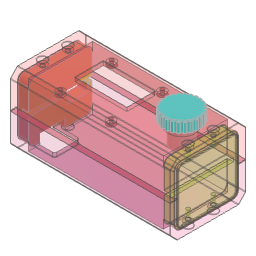
Gadget (Autodesk Fusion 360 design; units mm, degrees)
Autodesk Fusion 360 part; units mm, degrees
(part 1 of 2)
sketch "Top" plane through (0, 0, 0) normal (0, 0, 1) x (1, 0, 0) in component "Board"
  line L0 (35, 15) -> (-35, 15)
  line L1 (-35, 15) -> (-35, -15)
  line L2 (-35, -15) -> (35, -15)
  line L3 (35, -15) -> (35, 15)
  line L4 (35, 15) -> (-35, -15) construction
  line L5 (-35, 15) -> (35, -15) construction
  circle A0 centre (-33, -13) radius 1
  circle A1 centre (33, -13) radius 1
  circle A2 centre (-33, 13) radius 1
  circle A3 centre (33, 13) radius 1
  line L6 (6.5, -14.5) -> (-21, -14.5)
  line L7 (-21, -14.5) -> (-21, 13.3)
  line L8 (-21, 13.3) -> (6.5, 13.3)
  line L9 (6.5, 13.3) -> (6.5, -14.5)
  line L10 (6.5, -14.5) -> (-21, 13.3) construction
  line L11 (-21, -14.5) -> (6.5, 13.3) construction
  circle A4 centre (24, 1.5) radius 3
  line L12 (-21, 10.8) -> (6.5, 10.8)
  line L13 (15.5167, -1.5) -> (30.0322, -1.5) construction
  line L14 (21.3737, 2.95) -> (26.6263, 2.95)
  circle A5 centre (-19.25, -12.75) radius 1
  circle A6 centre (-19.25, -12.75) radius 1.75
  line L15 (-21, -0.6) -> (6.5, -0.6) construction
  line L16 (-7.25, -14.5) -> (-7.25, 13.3) construction
  circle A7 centre (4.75, -12.75) radius 1
  circle A8 centre (4.75, -12.75) radius 1.75
  circle A9 centre (-19.25, 11.55) radius 1.75
  circle A10 centre (-19.25, 11.55) radius 1
  circle A11 centre (4.75, 11.55) radius 1
  circle A12 centre (4.75, 11.55) radius 1.75
  line L17 (-21, -10.5) -> (6.5, -10.5)
  line L18 (-21, 9.3) -> (6.5, 9.3)
  point P0 (-7.25, -0.6)
  dimension "d1" = 70
  dimension "d2" = 30
  dimension "d3" = 2
  dimension "d4" = 2
  dimension "d5" = 2
  dimension "d8" = 66
  dimension "d9" = 26
  dimension "d10" = 27.5
  dimension "d11" = 27.8
  dimension "d12" = 14
  dimension "d13" = 0.5
  dimension "d14" = 6
  dimension "d15" = 13.5
  dimension "d16" = 11
  dimension "d29" = 2.5
  dimension "d36" = 4.45
  dimension "d40" = 2
  dimension "d41" = 3.5
  dimension "d42" = 4
  dimension "d43" = 4
  constraint horizontal L0
  constraint perpendicular L0 L1
  constraint parallel L0 L2
  constraint parallel L1 L3
  constraint coincident L4 origin
  constraint coincident L5 origin
  constraint horizontal L6
  constraint perpendicular L6 L7
  constraint parallel L6 L8
  constraint parallel L7 L9
  constraint coincident L10 P0
  constraint coincident L11 P0
  constraint coincident L7 L12.start
  constraint coincident L9 L12.end
  constraint perpendicular L9 L12
  constraint horizontal L13
  constraint tangent A4 L13
  constraint coincident A4 L14.start
  constraint coincident A4 L14.end
  constraint horizontal L14
  constraint concentric A5 A6
  constraint tangent L7 A6
  constraint tangent L6 A6
  constraint midpoint L7 L15.start
  constraint midpoint L9 L15.end
  constraint midpoint L6 L16.start
  constraint midpoint L8 L16.end
  constraint symmetric A5 L16 A7
  constraint symmetric A6 L16 A8
  constraint symmetric A5 L15 A10
  constraint symmetric A6 L15 A9
  constraint symmetric L15 A7 A11
  constraint symmetric L15 A8 A12
  constraint coincident L7 L17.start
  constraint coincident L9 L17.end
  constraint perpendicular L9 L17
  constraint coincident L7 L18.start
  constraint coincident L9 L18.end
  constraint perpendicular L9 L18
  measures "d1" distance of L1.end L2.end
  measures "d2" distance of L0.end L1.end
  measures "d3" diameter of A0
  measures "d4" distance of L1 A0.centre
  measures "d5" distance of L2 A0.centre
  measures "d10" distance of L7.end L8.end
  measures "d11" distance of L6.end L7.end
  measures "d12" distance of L1 L7
  measures "d13" distance of L2 L6
  measures "d14" diameter of A4
  measures "d15" distance of L0 A4.centre
  measures "d16" distance of L3 A4.centre
  measures "d29" distance of L7.end L12.start
  measures "d36" distance of L13 L14.end
  measures "d40" diameter of A5
  measures "d41" diameter of A6
  measures "d42" distance of L6.start L17.end
  measures "d43" distance of L8.end L18.end
extrude "Extrude1" add sketch "Top" along normal mid plane 1.6 contours L0 L1 L2 L3 | L6 L9 A8 | L6 L7 L9 A6 A8 L17 | A8 | L6 L7 A6 | A6 | L7 L9 L17 L18 | L7 L9 L12 A9 A12 L18 | L9 L12 A12 | L8 L9 A12 | L12 A11 A12 | L12 A11 A12 | L7 L12 A9 | L8 L12 A9 A12 | L12 A11 | L12 A11 | L7 L8 A9 | L12 A9 A10 | L12 A9 A10 | L12 A10 | L12 A10 | A4 L14 | A4 L14 | A5 | A7 makes body 1 in component "Board"
extrude "Extrude2" add sketch "Top" along normal blind 14.5 from surface at 0.8 contours L6 L9 A8 | L6 L7 L9 A6 A8 L17 | A8 | L6 L7 A6 | A6 | L7 L9 L17 L18 | L7 L9 L12 A9 A12 L18 | L9 L12 A12 | L8 L9 A12 | L12 A11 A12 | L12 A11 A12 | L7 L12 A9 | L8 L12 A9 A12 | L7 L8 A9 | L12 A9 A10 | L12 A9 A10 bodies 1 in component "Board"
extrude "Extrude4" cut sketch "Top" along normal up to surface (10.7 mm away) from surface at 0.8 contours L6 L9 A8 | L6 L7 L9 A6 A8 L17 | A8 | L6 L7 A6 | A6 | L7 L9 L17 L18 | L7 L9 L12 A9 A12 L18 | L12 A11 A12 | L12 A11 | L12 A9 A10 | L12 A10 | A5 | A7 picked at (5.7851, 10.4689) picked at (4.9322, 10.7708) picked at (-18.2149, 10.4689) picked at (-19.4322, 10.7708) bodies 1 in component "Board"
extrude "Extrude7" cut sketch "Top" along normal through all from surface at 13.5 contours L6 L9 A8 | L6 L7 L9 A6 A8 L17 | A8 | L6 L7 A6 | A6 | L7 L9 L12 A9 A12 L18 | L9 L12 A12 | L8 L9 A12 | L12 A11 A12 | L12 A11 A12 | L7 L12 A9 | L8 L12 A9 A12 | L7 L8 A9 | L12 A9 A10 | L12 A9 A10 bodies 1 in component "Board"
extrude "Extrude5" add sketch "Top" along normal blind 14.1 from surface at 0.8 contours A4 L14 | A4 L14 bodies 1 in component "Board"
extrude "Extrude6" cut sketch "Top" against normal blind 10 from surface at 14.9 contours A4 L14 picked at (23.2953, 3.1762) bodies 1 in component "Board"
sketch "Bottom" plane through (0, 0, 0) normal (0, 0, 1) x (1, 0, 0) in component "Board"
  line L0 (-35, -15) -> (35, -15) construction
  circle A0 centre (-33, -13) radius 1 construction
  line L1 (-35, 15) -> (-35, -15) construction
  line L2 (35, 15) -> (-35, 15) construction
  circle A1 centre (-33, 13) radius 1 construction
  circle A2 centre (33, 13) radius 1 construction
  line L3 (35, -15) -> (35, 15) construction
  circle A3 centre (33, -13) radius 1 construction
  line L4 (31.8, 12.7) -> (12.6, 12.7)
  line L5 (12.6, 12.7) -> (12.6, -13.5)
  line L6 (12.6, -13.5) -> (31.8, -13.5)
  line L7 (31.8, -13.5) -> (31.8, 12.7)
  line L8 (31.8, 12.7) -> (12.6, -13.5) construction
  line L9 (12.6, 12.7) -> (31.8, -13.5) construction
  line L10 (10.4, 14.8) -> (-2.8, 14.8)
  line L11 (-2.8, 14.8) -> (-2.8, -12.7)
  line L12 (-2.8, -12.7) -> (10.4, -12.7)
  line L13 (10.4, -12.7) -> (10.4, 14.8)
  line L14 (10.4, 14.8) -> (-2.8, -12.7) construction
  line L15 (-2.8, 14.8) -> (10.4, -12.7) construction
  line L16 (-10.8, 5.08) -> (-32, 5.08)
  line L17 (-32, 5.08) -> (-32, -12.7)
  line L18 (-32, -12.7) -> (-10.8, -12.7)
  line L19 (-10.8, -12.7) -> (-10.8, 5.08)
  line L20 (-10.8, 5.08) -> (-32, -12.7) construction
  line L21 (-32, 5.08) -> (-10.8, -12.7) construction
  line L22 (-25.9, 0.69) -> (-33.4, 0.69)
  line L23 (-33.4, 0.69) -> (-33.4, -8.31)
  line L24 (-33.4, -8.31) -> (-25.9, -8.31)
  line L25 (-25.9, -8.31) -> (-25.9, 0.69)
  line L26 (-25.9, 0.69) -> (-33.4, -8.31) construction
  line L27 (-33.4, 0.69) -> (-25.9, -8.31) construction
  line L28 (-29.65, -3.81) -> (-21.4, -3.81) construction
  line L29 (-31.5, 13) -> (-38.5, 13)
  line L30 (-38.5, 13) -> (-38.5, 4)
  line L31 (-38.5, 4) -> (-31.5, 4)
  line L32 (-31.5, 4) -> (-31.5, 13)
  line L33 (-31.5, 13) -> (-38.5, 4) construction
  line L34 (-38.5, 13) -> (-31.5, 4) construction
  point P0 (22.2, -0.4)
  point P1 (3.8, 1.05)
  point P2 (-21.4, -3.81)
  point P3 (-29.65, -3.81)
  point P4 (-35, 8.5)
  dimension "d46" = 19.2
  dimension "d47" = 26.2
  dimension "d48" = 1.5
  dimension "d49" = 3.2
  dimension "d50" = 13.2
  dimension "d51" = 27.5
  dimension "d53" = 2.2
  dimension "d54" = 8
  dimension "d55" = 17.78
  dimension "d56" = 21.2
  dimension "d57" = 7.5
  dimension "d58" = 9
  dimension "d59" = 1.4
  dimension "d70" = 63.8
  dimension "d378" = 7
  dimension "d379" = 9
  dimension "d400" = 2.3
  dimension "d401" = 2
  dimension "d402" = 2.3
  constraint horizontal L4
  constraint perpendicular L4 L5
  constraint parallel L4 L6
  constraint parallel L5 L7
  constraint coincident L8 P0
  constraint coincident L9 P0
  constraint horizontal L10
  constraint perpendicular L10 L11
  constraint parallel L10 L12
  constraint parallel L11 L13
  constraint coincident L14 P1
  constraint coincident L15 P1
  constraint horizontal L16
  constraint perpendicular L16 L17
  constraint parallel L16 L18
  constraint parallel L17 L19
  constraint coincident L20 P2
  constraint coincident L21 P2
  constraint horizontal L22
  constraint perpendicular L22 L23
  constraint parallel L22 L24
  constraint parallel L23 L25
  constraint coincident L26 P3
  constraint coincident L27 P3
  constraint coincident P3 L28.start
  constraint coincident P2 L28.end
  constraint perpendicular L17 L28
  constraint horizontal L29
  constraint perpendicular L29 L30
  constraint parallel L29 L31
  constraint parallel L30 L32
  constraint coincident L33 P4
  constraint coincident L34 P4
  constraint coincident L1 P4
  measures "d46" distance of L5.end L6.end
  measures "d47" distance of L4.end L5.end
  measures "d48" distance of L0 L6
  measures "d49" distance of L3 L7
  measures "d50" distance of L11.end L12.end
  measures "d51" distance of L10.end L11.end
  measures "d53" distance of L5 L13
  measures "d54" distance of L11 L19
  measures "d55" distance of L16.end L17.end
  measures "d56" distance of L17.end L18.end
  measures "d57" distance of L23.end L24.end
  measures "d58" distance of L22.end L23.end
  measures "d59" distance of L17 L22.end
  measures "d70" horizontal distance of L4.start L16.end
  measures "d378" distance of L30.end L31.end
  measures "d379" distance of L29.end L30.end
  measures "d400" distance of L0 L18
  measures "d401" distance of L2 L29
  measures "d402" distance of L0 L12
extrude "Extrude8" add sketch "Bottom" against normal blind 4 from surface at -0.8 contours L16 L17 L31 L32 | L16 L17 L29 L30 L31 L32 bodies 1 in component "Board"
extrude "Extrude9" add sketch "Bottom" against normal blind 13.5 from surface at -0.8 contours L16 L17 L18 L19 L22 L24 L25 L31 L32 | L16 L17 L31 L32 | L17 L22 L24 L25 bodies 1 in component "Board"
extrude "Extrude10" add sketch "Bottom" against normal blind 3.2 from surface at -12.7 contours L17 L22 L23 L24 | L17 L22 L24 L25 bodies 1 in component "Board"
extrude "Extrude11" add sketch "Bottom" against normal blind 13.9 from surface at -0.8 contours L10 L11 L12 L13 bodies 1 in component "Board"
extrude "Extrude12" add sketch "Bottom" against normal blind 13.9 from surface at -0.8 contours L4 L5 L6 L7 bodies 1 in component "Board"
sketch "Sketch1" plane through (0, 0, 0) normal (1, 0, 0) x (0, 1, 0) in component "Right"
  line L0 (12, -13.9) -> (-12, -13.9)
  line L1 (-15, -10.9) -> (-15, 10.9)
  line L2 (-12, 13.9) -> (12, 13.9)
  line L3 (15, 10.9) -> (15, -10.9)
  line L4 (15, -13.9) -> (-15, 13.9) construction
  line L5 (-15, -13.9) -> (15, 13.9) construction
  arc A0 (-12, 13.9) -> (-15, 10.9) centre (-12, 10.9) ccw
  arc A1 (15, 10.9) -> (12, 13.9) centre (12, 10.9) ccw
  arc A2 (12, -13.9) -> (15, -10.9) centre (12, -10.9) ccw
  arc A3 (-15, -10.9) -> (-12, -13.9) centre (-12, -10.9) ccw
  line L6 (-15, -0.9) -> (15, -0.9)
  line L7 (-15, 0.9) -> (15, 0.9)
  arc A4 (13.9, 10.9) -> (12, 12.8) centre (12, 10.9) ccw
  line L8 (-12, 12.8) -> (12, 12.8)
  arc A5 (-12, 12.8) -> (-13.9, 10.9) centre (-12, 10.9) ccw
  line L9 (-13.9, -10.9) -> (-13.9, 10.9)
  arc A6 (-13.9, -10.9) -> (-12, -12.8) centre (-12, -10.9) ccw
  line L10 (12, -12.8) -> (-12, -12.8)
  arc A7 (12, -12.8) -> (13.9, -10.9) centre (12, -10.9) ccw
  line L11 (13.9, 10.9) -> (13.9, -10.9)
  dimension "d192" = 30
  dimension "d193" = 27.8
  dimension "d194" = 3
  dimension "d209" = 1.1
  dimension "d393" = 1.8
  dimension "d394" = 0.9
  constraint horizontal L0
  constraint perpendicular L0 L1
  constraint parallel L0 L2
  constraint parallel L1 L3
  constraint coincident L4 origin
  constraint coincident L5 origin
  constraint coincident L4.end L1
  constraint coincident L4.end L2
  constraint tangent L1 A0
  constraint tangent L2 A0
  constraint coincident L5.end L3
  constraint coincident L5.end L2
  constraint tangent L3 A1
  constraint tangent L2 A1
  constraint equal A0 A1
  constraint coincident L4.start L0
  constraint coincident L4.start L3
  constraint tangent L0 A2
  constraint tangent L3 A2
  constraint equal A0 A2
  constraint coincident L5.start L0
  constraint coincident L5.start L1
  constraint tangent L0 A3
  constraint tangent L1 A3
  constraint equal A0 A3
  constraint coincident L1 L6.start
  constraint coincident L3 L6.end
  constraint perpendicular L3 L6
  constraint coincident L1 L7.start
  constraint coincident L3 L7.end
  constraint perpendicular L3 L7
  measures "d192" distance of L4.end L5.end
  measures "d193" distance of L5.start L4.end
  measures "d194" radius of A0
  measures "d393" distance of L6.end L7.end
  measures "d394" distance of origin L6
extrude "Extrude1'" add sketch "Sketch1" along normal blind 6 from surface at 32 separate body makes body 2 in component "Right"
extrude "Extrude2'" cut sketch "Sketch1" along normal blind 35 contours L3 L6 L7 L11 | L1 L6 L7 L9 | L6 L7 L9 L11 bodies 2 in component "Right"
extrude "Extrude5'" cut sketch "Sketch1" against normal blind 1 from surface at 38 contours L0 L1 L3 A2 A3 L6 L9 A6 L10 A7 L11 | L3 L6 L7 L11 | L1 L6 L7 L9 | L1 L2 L3 A0 A1 L7 A4 L8 A5 L9 L11 bodies 2 in component "Right"
sketch "Sketch2" plane through (0, 0, 13.9) normal (0, 0, 1) x (-1, 0, 0) in component "Right"
  line L0 (-32, -12) -> (-32, 12)
  line L1 (-32, 12) -> (-37, 12)
  line L2 (-37, -12) -> (-32, -12)
  line L3 (0, 0) -> (-32, 0) construction
  line L4 (-32, 0) -> (-37, 0) construction
  line L5 (-34.5, 0) -> (-34.5, -6) construction
  circle A0 centre (-34.5, -6) radius 0.875
  circle A1 centre (-34.5, 6) radius 0.875
  line L6 (-37, 12) -> (-37, -12)
  dimension "d202" = 6
  dimension "d203" = 1.75
  constraint coincident L3.start origin
  constraint midpoint L0 L3.end
  constraint midpoint L4 L5.start
  constraint perpendicular L4 L5
  constraint coincident L5.end A0.centre
  constraint symmetric L4 A0 A1
  constraint midpoint L4.end L6
  measures "d202" distance of L5.start L5.end
  measures "d203" diameter of A0
extrude "Extrude3" cut sketch "Sketch2" against normal blind 4 contours A0 | A1 bodies 2 in component "Right"
extrude "Extrude4'" cut sketch "Sketch2" along normal blind 4 from surface at -27.8 contours A0 | A1 bodies 2 in component "Right"
chamfer "Chamfer1" distance 0.2 angle 45 8 edges at (37, 0, 13.9) (37, 14.1213, 13.0213) (37, 15, 0) (37, 14.1213, -13.0213) (37, 0, -13.9) (37, -14.1213, -13.0213) (37, -15, 0) (37, -14.1213, 13.0213) 2 faces at (32, -4, -5.2333) (32, -4, 5.2333) on bodies 2 in component "Right"
sketch "Sketch1 (2)" plane through (0, 0, 0) normal (1, 0, 0) x (0, 1, 0) in component "Left"
  line L0 (12, -13.9) -> (-12, -13.9)
  line L1 (-15, -10.9) -> (-15, 10.9)
  line L2 (-12, 13.9) -> (12, 13.9)
  line L3 (15, 10.9) -> (15, -10.9)
  line L4 (15, -13.9) -> (-15, 13.9) construction
  line L5 (-15, -13.9) -> (15, 13.9) construction
  arc A0 (-12, 13.9) -> (-15, 10.9) centre (-12, 10.9) ccw
  arc A1 (15, 10.9) -> (12, 13.9) centre (12, 10.9) ccw
  arc A2 (12, -13.9) -> (15, -10.9) centre (12, -10.9) ccw
  arc A3 (-15, -10.9) -> (-12, -13.9) centre (-12, -10.9) ccw
  arc A4 (13.9, 10.9) -> (12, 12.8) centre (12, 10.9) ccw
  line L6 (-12, 12.8) -> (12, 12.8)
  arc A5 (-12, 12.8) -> (-13.9, 10.9) centre (-12, 10.9) ccw
  line L7 (-13.9, -10.9) -> (-13.9, 10.9)
  arc A6 (-13.9, -10.9) -> (-12, -12.8) centre (-12, -10.9) ccw
  line L8 (12, -12.8) -> (-12, -12.8)
  arc A7 (12, -12.8) -> (13.9, -10.9) centre (12, -10.9) ccw
  line L9 (13.9, 10.9) -> (13.9, -10.9)
  line L10 (-15, -0.9) -> (15, -0.9)
  line L11 (-15, 0.9) -> (15, 0.9)
  line L12 (2.19, -18.3) -> (-9.81, -18.3)
  line L13 (-9.81, -18.3) -> (-9.81, -10.3)
  line L14 (-9.81, -10.3) -> (2.19, -10.3)
  line L15 (2.19, -10.3) -> (2.19, -18.3)
  line L16 (2.19, -18.3) -> (-9.81, -10.3) construction
  line L17 (-9.81, -18.3) -> (2.19, -10.3) construction
  line L18 (4, -0.8) -> (13, -0.8)
  line L19 (13, -0.8) -> (13, -4.8)
  line L20 (13, -4.8) -> (4, -4.8)
  line L21 (4, -4.8) -> (4, -0.8)
  line L22 (3, -5.8) -> (3, 0.2)
  line L23 (3, 0.2) -> (14, 0.2)
  line L24 (14, 0.2) -> (14, -5.8)
  line L25 (14, -5.8) -> (3, -5.8)
  line L26 (-8.31, -12.7) -> (0.69, -12.7)
  line L27 (0.69, -12.7) -> (0.69, -15.9)
  line L28 (0.69, -15.9) -> (-8.31, -15.9)
  line L29 (-8.31, -15.9) -> (-8.31, -12.7)
  line L30 (-3.81, -14.3) -> (-8.31, -14.3) construction
  line L31 (-3.81, -14.3) -> (-3.81, -15.9) construction
  point P0 (-3.81, -14.3)
  dimension "d214" = 30
  dimension "d215" = 27.8
  dimension "d216" = 3
  dimension "d217" = 1.1
  dimension "d218" = 0.9
  dimension "d231" = 12
  dimension "d232" = 8
  dimension "d381" = -1
  dimension "d395" = 1.8
  constraint horizontal L0
  constraint perpendicular L0 L1
  constraint parallel L0 L2
  constraint parallel L1 L3
  constraint coincident L4 origin
  constraint coincident L5 origin
  constraint coincident L4.end L1
  constraint coincident L4.end L2
  constraint tangent L1 A0
  constraint tangent L2 A0
  constraint coincident L5.end L3
  constraint coincident L5.end L2
  constraint tangent L3 A1
  constraint tangent L2 A1
  constraint equal A0 A1
  constraint coincident L4.start L0
  constraint coincident L4.start L3
  constraint tangent L0 A2
  constraint tangent L3 A2
  constraint equal A0 A2
  constraint coincident L5.start L0
  constraint coincident L5.start L1
  constraint tangent L0 A3
  constraint tangent L1 A3
  constraint equal A0 A3
  constraint coincident L1 L10.start
  constraint coincident L3 L10.end
  constraint perpendicular L3 L10
  constraint coincident L1 L11.start
  constraint coincident L3 L11.end
  constraint perpendicular L3 L11
  constraint horizontal L12
  constraint perpendicular L12 L13
  constraint parallel L12 L14
  constraint parallel L13 L15
  constraint coincident L16 P0
  constraint coincident L17 P0
  constraint coincident P0 L30.start
  constraint coincident L29 L30.end
  constraint perpendicular L29 L30
  constraint midpoint L29 L30.end
  constraint coincident L28 L31.end
  constraint perpendicular L28 L31
  constraint midpoint L28 L31.end
  measures "d214" distance of L4.end L5.end
  measures "d215" distance of L5.start L4.end
  measures "d216" radius of A0
  measures "d218" vertical distance of origin L10.end
  measures "d231" distance of L13.end L14.end
  measures "d232" distance of L12.end L13.end
  measures "d395" distance of L10.end L11.end
extrude "Extrude1''" add sketch "Sketch1 (2)" against normal blind 6 from surface at -32 separate body contours L0 L3 A2 L8 A7 L9 L10 L15 L24 L25 | L7 A6 L8 A7 L9 L10 L13 L14 L15 L22 L25 | L3 L9 L10 L11 L23 L24 | L1 L2 L3 A0 A1 A4 L6 A5 L7 L9 L11 | L9 L10 L24 L25 | L9 L10 L23 L24 | L0 L1 A3 L7 A6 L8 L10 L13 | A4 L6 A5 L7 L9 L11 | L7 L9 L10 L11 L22 L23 | L9 L10 L18 L19 L21 L22 L23 | L9 L10 L19 L20 L21 L22 L25 | L1 L7 L10 L11 makes body 3 in component "Left"
extrude "Extrude2''" cut sketch "Sketch1 (2)" against normal blind 35 contours L3 L9 L10 L11 L23 L24 | L9 L10 L23 L24 | L7 L9 L10 L11 L22 L23 | L9 L10 L18 L19 L21 L22 L23 | L1 L7 L10 L11 | L10 L18 L19 L21 bodies 3 in component "Left"
extrude "Extrude3'" cut sketch "Sketch1 (2)" along normal blind 1 from surface at -38 contours L0 L3 A2 L8 A7 L9 L10 L15 L24 L25 | L0 L8 L15 L27 | L0 L8 L27 L29 | L3 L9 L10 L11 L23 L24 | L0 L8 L13 L29 | L1 L2 L3 A0 A1 A4 L6 A5 L7 L9 L11 | L9 L10 L24 L25 | L9 L10 L23 L24 | L0 L1 A3 L7 A6 L8 L10 L13 | L1 L7 L10 L11 bodies 3 in component "Left"
extrude "Extrude7'" cut sketch "Sketch1 (2)" along normal blind 1 from surface at -38 contours L9 L10 L24 L25 | L9 L10 L23 L24 | L9 L10 L18 L19 L21 L22 L23 | L9 L10 L19 L20 L21 L22 L25 bodies 3 in component "Left"
fillet "Fillet1" radius 1 2 edges at (-37.5, 3, 0.2) (-37.5, 3, -5.8) on bodies 3 in component "Left"
fillet "Fillet2" radius 1 5 edges at (-37, 8.95, -5.8) (-37, 3.2929, -5.5071) (-37, 3, -2.8) (-37, 3.2929, -0.0929) (-37, 8.95, 0.2) on bodies 3 in component "Left"
sketch "Sketch2 (2)" plane through (0, 0, 13.9) normal (0, 0, 1) x (-1, 0, 0) in component "Left"
  line L0 (37, -12) -> (37, 12)
  line L1 (37, 12) -> (32, 12)
  line L2 (32, 12) -> (32, -12)
  line L3 (32, -12) -> (37, -12)
  line L4 (0, 0) -> (32, 0) construction
  line L5 (32, 0) -> (37, 0) construction
  line L6 (34.5, 0) -> (34.5, -6) construction
  circle A0 centre (34.5, -6) radius 0.875
  circle A1 centre (34.5, 6) radius 0.875
  dimension "d235" = 5
  dimension "d236" = 6
  dimension "d237" = 1.75
  constraint coincident L4.start origin
  constraint midpoint L2 L4.end
  constraint perpendicular L0 L5
  constraint midpoint L5 L6.start
  constraint perpendicular L5 L6
  constraint coincident L6.end A0.centre
  constraint symmetric L5 A0 A1
  measures "d235" distance of L4.end L5.end
  measures "d236" distance of L6.start L6.end
  measures "d237" diameter of A0
extrude "Extrude4''" cut sketch "Sketch2 (2)" against normal blind 4 contours A0 | A1 bodies 3 in component "Left"
extrude "Extrude5''" cut sketch "Sketch2 (2)" along normal blind 4 from surface at -27.8 contours A0 bodies 3 in component "Left"
chamfer "Chamfer1'" distance 0.2 angle 45 9 edges at (-37, -14.1213, 13.0213) (-37, 0, 13.9) (-37, 14.1213, 13.0213) (-37, 15, 0) (-37, 14.1213, -13.0213) (-37, 7.095, -13.9) (-37, -10.905, -13.9) (-37, -14.1213, -13.0213) (-37, -15, 0) 2 faces at (-32, -4, 5.2333) (-32, -6.9367, -4.0333) on bodies 3 in component "Left"
sketch "Sketch1 (3)" plane through (0, 0, 0) normal (1, 0, 0) x (0, 1, 0) in component "Bottom"
  line L0 (-12, -13.9) -> (12, -13.9) construction
  line L1 (15, -10.9) -> (15, 10.9) construction
  line L2 (12, 13.9) -> (-12, 13.9) construction
  line L3 (-15, 10.9) -> (-15, -10.9) construction
  line L4 (-15, -13.9) -> (15, 13.9) construction
  line L5 (15, -13.9) -> (-15, 13.9) construction
  arc A0 (15, 10.9) -> (12, 13.9) centre (12, 10.9) ccw construction
  arc A1 (-12, 13.9) -> (-15, 10.9) centre (-12, 10.9) ccw construction
  arc A2 (-15, -10.9) -> (-12, -13.9) centre (-12, -10.9) ccw construction
  arc A3 (12, -13.9) -> (15, -10.9) centre (12, -10.9) ccw construction
  line L6 (-12, -13.1) -> (12, -13.1)
  arc A4 (12, -13.1) -> (14.2, -10.9) centre (12, -10.9) ccw
  line L7 (14.2, -10.9) -> (14.2, 10.9)
  arc A5 (14.2, 10.9) -> (12, 13.1) centre (12, 10.9) ccw
  line L8 (12, 13.1) -> (-12, 13.1)
  arc A6 (-12, 13.1) -> (-14.2, 10.9) centre (-12, 10.9) ccw
  line L9 (-14.2, 10.9) -> (-14.2, -10.9)
  arc A7 (-14.2, -10.9) -> (-12, -13.1) centre (-12, -10.9) ccw
  line L10 (-12, -14.1) -> (12, -14.1)
  arc A8 (12, -14.1) -> (15.2, -10.9) centre (12, -10.9) ccw
  line L11 (15.2, -10.9) -> (15.2, 10.9)
  arc A9 (15.2, 10.9) -> (12, 14.1) centre (12, 10.9) ccw
  line L12 (12, 14.1) -> (-12, 14.1)
  arc A10 (-12, 14.1) -> (-15.2, 10.9) centre (-12, 10.9) ccw
  line L13 (-15.2, 10.9) -> (-15.2, -10.9)
  arc A11 (-15.2, -10.9) -> (-12, -14.1) centre (-12, -10.9) ccw
  line L14 (-18, 10.9) -> (-18, -10.9)
  arc A12 (-18, -10.9) -> (-12, -16.9) centre (-12, -10.9) ccw construction
  line L15 (-12, -16.9) -> (12, -16.9)
  arc A13 (12, -16.9) -> (18, -10.9) centre (12, -10.9) ccw construction
  line L16 (18, -10.9) -> (18, 10.9)
  arc A14 (18, 10.9) -> (12, 16.9) centre (12, 10.9) ccw
  line L17 (12, 16.9) -> (-12, 16.9)
  arc A15 (-12, 16.9) -> (-18, 10.9) centre (-12, 10.9) ccw
  line L18 (18, 0) -> (-18, 0)
  line L19 (2.19, -18.3) -> (-9.81, -18.3)
  line L20 (2.19, -10.3) -> (2.19, -18.3)
  line L21 (-9.81, -18.3) -> (-9.81, -10.3)
  line L22 (-9.81, -10.3) -> (2.19, -10.3)
  line L23 (-15.2, -10.9) -> (-15.2, -15)
  line L24 (-15.2, -15) -> (15.2, -15)
  line L25 (15.2, -15) -> (15.2, -10.9)
  line L26 (-14.5804, -16.9) -> (-18, -13.2912)
  line L27 (-18, -13.2912) -> (-18, -10.9)
  line L28 (-14.5804, -16.9) -> (-12, -16.9)
  line L29 (-15, -13.9) -> (-16.2902, -15.0956) construction
  line L30 (0, 0) -> (0, -13.1) construction
  line L31 (14.5804, -16.9) -> (12, -16.9)
  line L32 (14.5804, -16.9) -> (18, -13.2912)
  line L33 (18, -13.2912) -> (18, -10.9)
  dimension "d244" = 30
  dimension "d245" = 27.8
  dimension "d246" = 3
  dimension "d247" = 3
  dimension "d248" = 3
  dimension "d249" = 3
  dimension "d250" = 0.2
  dimension "d251" = -0.8
  dimension "d252" = 3
  dimension "d284" = 15
  constraint horizontal L0
  constraint perpendicular L0 L1
  constraint parallel L0 L2
  constraint parallel L1 L3
  constraint coincident L4 L30.start
  constraint coincident L5 L30.start
  constraint coincident L30.start origin
  constraint coincident L4.end L2
  constraint coincident L4.end L1
  constraint tangent L2 A0
  constraint tangent L1 A0
  constraint coincident L5.end L2
  constraint coincident L5.end L3
  constraint tangent L2 A1
  constraint tangent L3 A1
  constraint coincident L4.start L0
  constraint coincident L4.start L3
  constraint tangent L0 A2
  constraint tangent L3 A2
  constraint coincident L5.start L0
  constraint coincident L5.start L1
  constraint tangent L0 A3
  constraint tangent L1 A3
  constraint midpoint L16 L18.start
  constraint midpoint L14 L18.end
  constraint perpendicular L14 L18
  constraint tangent A11 L23
  constraint parallel L13 L23
  constraint perpendicular L20 L24
  constraint perpendicular L24 L25
  constraint parallel L15 L28
  constraint parallel L14 L27
  constraint tangent A12 L26
  constraint coincident L26 L29.end
  constraint parallel L4 L29
  constraint midpoint L26 L29.end
  constraint midpoint L6 L30.end
  constraint perpendicular L6 L30
  constraint symmetric L14.end L30 A13.end
  constraint symmetric A12.end L30 L15.end
  constraint symmetric L26.start L30 L31.start
  constraint symmetric L26.end L30 L32.end
  measures "d244" distance of L4.end L5.end
  measures "d245" distance of L5.start L4.end
  measures "d246" radius of A0
  measures "d247" radius of A1
  measures "d248" radius of A2
  measures "d249" radius of A3
  measures "d284" vertical distance of L18.end L23.end
extrude "Extrude1'''" add sketch "Sketch1 (3)" along normal mid plane 76 separate body contours L6 L9 A7 L10 L13 A11 L18 L21 | L6 L10 L20 L21 | L6 A4 L7 L10 A8 L11 L18 L20 | L10 A11 L21 L23 L24 | L10 L20 L21 L24 | L10 A8 L20 L24 L25 | L15 L20 L21 L24 | L13 L14 L15 L18 L21 L23 L24 L26 L27 L28 | L11 L15 L16 L18 L20 L24 L25 L31 L32 L33 makes body 4 in component "Bottom"
extrude "Extrude3''" cut sketch "Sketch1 (3)" along normal mid plane 74.4 contours L6 L9 A7 L10 L13 A11 L18 L21 | L6 L10 L20 L21 | L6 A4 L7 L10 A8 L11 L18 L20 bodies 4 in component "Bottom"
extrude "Extrude7''" cut sketch "Sketch1 (3)" along normal mid plane 64 contours L10 A11 L21 L23 L24 | L10 L20 L21 L24 | L10 A8 L20 L24 L25 bodies 4 in component "Bottom"
extrude "Extrude4'''" cut sketch "Sketch1 (2)" along normal blind 13 from surface at -38 contours L0 L12 L13 L15 L27 L28 L29 | L0 L8 L15 L27 | L0 L27 L28 L29 | L0 L8 L27 L29 | L8 L13 L14 L15 L26 L27 L29 | L0 L8 L13 L29 | L8 L26 L27 L29 bodies 4 in component "Bottom"
fillet "Fillet1'" radius 1 2 edges at (-25, 2.19, -15.95) (-25, -9.81, -15.95) on bodies 4 in component "Bottom"
sketch "Sketch2 (3)" plane through (0, 0, 0) normal (0, 0, 1) x (1, 0, 0) in component "Bottom"
  circle A0 centre (-34.5, -6) radius 1
  circle A1 centre (-34.5, 6) radius 1
  circle A2 centre (34.5, 6) radius 1
  circle A3 centre (34.5, -6) radius 1
  circle A4 centre (-34.5, -6) radius 2
  circle A5 centre (-34.5, 6) radius 2
  circle A6 centre (34.5, 6) radius 2
  circle A7 centre (34.5, -6) radius 2
  point P0 (-34.5, -6)
  point P1 (-34.5, 6)
  point P2 (34.5, 6)
  point P3 (34.5, -6)
  dimension "d271" = 2
  dimension "d272" = 2
  dimension "d273" = 2
  dimension "d274" = 2
  dimension "d275" = 4
  dimension "d276" = 4
  dimension "d277" = 4
  dimension "d278" = 4
  constraint coincident P0 A0.centre
  constraint coincident P1 A1.centre
  constraint coincident P2 A2.centre
  constraint coincident P3 A3.centre
  constraint concentric A2 A6
  constraint concentric A3 A7
  measures "d271" diameter of A0
  measures "d272" diameter of A1
  measures "d273" diameter of A2
  measures "d274" diameter of A3
  measures "d275" diameter of A4
  measures "d276" diameter of A5
  measures "d277" diameter of A6
  measures "d278" diameter of A7
extrude "Extrude5'''" cut sketch "Sketch2 (3)" against normal through all contours A1 | A2 | A3 bodies 4 in component "Bottom"
extrude "Extrude6'" cut sketch "Sketch2 (3)" along normal blind 2 from surface at -16.9 contours A5 | A6 | A7 bodies 4 in component "Bottom"
chamfer "Chamfer5" distance 0.5 distance2 1 3 edges at (33.5677, -5.6384, -14.9) (33.5677, 6.3616, -14.9) (-35.4323, 6.3616, -14.9) measured on face at (35.1982, -5.2841, -14.3667) measured on face at (33.734, 6.6428, -14.3667) measured on face at (-33.7029, 6.6038, -14.6333) on bodies 4 in component "Bottom"
chamfer "Chamfer6" distance 0.2 distance2 0.2 6 faces at (-8.4707, 10.3866, -16.9) (-38, -16.7333, -8.0637) (-38, 16.7333, -8.0637) (38, -4, -15.6333) (12.6667, 16.8601, -14.4941) (12.6667, -16.8601, -14.4941) on bodies 4 in component "Bottom"
sketch "Sketch1 (4)" plane through (0, 0, 0) normal (1, 0, 0) x (0, 1, 0) in component "Top"
  arc A0 (-12, 14.1) -> (-15.2, 10.9) centre (-12, 10.9) ccw
  arc A1 (15, 10.9) -> (12, 13.9) centre (12, 10.9) ccw construction
  line L0 (-15.2, 10.9) -> (-15.2, -10.9)
  line L1 (-15, 10.9) -> (-15, -10.9) construction
  line L2 (12, 14.1) -> (-12, 14.1)
  line L3 (12, 13.9) -> (-12, 13.9) construction
  line L4 (15, -13.9) -> (-15, 13.9) construction
  arc A2 (15.2, 10.9) -> (12, 14.1) centre (12, 10.9) ccw
  line L5 (-15, -13.9) -> (15, 13.9) construction
  line L6 (15.2, -10.9) -> (15.2, 10.9)
  arc A3 (-12, 13.9) -> (-15, 10.9) centre (-12, 10.9) ccw construction
  line L7 (15, -10.9) -> (15, 10.9) construction
  line L8 (18, 0) -> (-18, 0)
  line L9 (-12, -13.9) -> (12, -13.9) construction
  arc A4 (12, -13.9) -> (15, -10.9) centre (12, -10.9) ccw construction
  line L10 (-12, -14.1) -> (12, -14.1)
  arc A5 (12, -14.1) -> (15.2, -10.9) centre (12, -10.9) ccw
  arc A6 (-15.2, -10.9) -> (-12, -14.1) centre (-12, -10.9) ccw
  arc A7 (-15, -10.9) -> (-12, -13.9) centre (-12, -10.9) ccw construction
  line L11 (-14.5804, 16.9) -> (-12, 16.9)
  line L12 (-18, 13.2912) -> (-18, 10.9)
  line L13 (-15.2, 15) -> (15.2, 15)
  line L14 (15.2, 15) -> (15.2, 10.9)
  line L15 (-15.2, 10.9) -> (-15.2, 15)
  line L16 (0, 0) -> (0, 12.2) construction
  line L17 (14.5804, 16.9) -> (12, 16.9)
  line L18 (18, 13.2912) -> (18, 10.9)
  line L19 (-15, 13.9) -> (-16.2902, 15.0956) construction
  line L20 (-18, 13.2912) -> (-14.5804, 16.9)
  line L21 (18, 13.2912) -> (14.5804, 16.9)
  line L22 (-14.2, 10.9) -> (-14.2, -10.9)
  arc A8 (-14.2, -10.9) -> (-12, -13.1) centre (-12, -10.9) ccw
  line L23 (-12, -13.1) -> (12, -13.1)
  arc A9 (12, -13.1) -> (14.2, -10.9) centre (12, -10.9) ccw
  line L24 (14.2, -10.9) -> (14.2, 10.9)
  arc A10 (14.2, 10.9) -> (12, 13.1) centre (12, 10.9) ccw
  line L25 (12, 13.1) -> (-12, 13.1)
  arc A11 (-12, 13.1) -> (-14.2, 10.9) centre (-12, 10.9) ccw
  line L26 (-18, 10.9) -> (-18, -10.9)
  arc A12 (-18, -10.9) -> (-12, -16.9) centre (-12, -10.9) ccw
  line L27 (-12, -16.9) -> (12, -16.9)
  arc A13 (12, -16.9) -> (18, -10.9) centre (12, -10.9) ccw
  line L28 (18, -10.9) -> (18, 10.9)
  arc A14 (18, 10.9) -> (12, 16.9) centre (12, 10.9) ccw construction
  line L29 (12, 16.9) -> (-12, 16.9)
  arc A15 (-12, 16.9) -> (-18, 10.9) centre (-12, 10.9) ccw construction
  line L30 (12, 18) -> (-12, 18)
  arc A16 (-12, 18) -> (-18, 12) centre (-12, 12) ccw construction
  arc A17 (18, 12) -> (12, 18) centre (12, 12) ccw construction
  line L31 (-18, 14.3095) -> (-18, 12)
  line L32 (-18, 14.3095) -> (-14.6648, 18)
  line L33 (-14.6648, 18) -> (-12, 18)
  line L34 (14.6648, 18) -> (12, 18)
  line L35 (18, 14.3095) -> (14.6648, 18)
  line L36 (18, 14.3095) -> (18, 12)
  line L37 (-15.2, 12.5) -> (-18, 12.5)
  dimension "d292" = 0.2
  dimension "d295" = 30
  dimension "d296" = 27.8
  dimension "d297" = 3
  dimension "d298" = 3
  dimension "d299" = 3
  dimension "d300" = 3
  dimension "d303" = -0.8
  dimension "d304" = 15
  dimension "d305" = 3
  dimension "d336" = 12.5
  constraint horizontal L9
  constraint perpendicular L7 L9
  constraint parallel L3 L9
  constraint parallel L1 L7
  constraint coincident L16.start L5
  constraint coincident L16.start L4
  constraint coincident L16.start origin
  constraint coincident L5.end L3
  constraint coincident L5.end L7
  constraint tangent A1 L3
  constraint tangent A1 L7
  constraint coincident L4.end L3
  constraint coincident L4.end L1
  constraint tangent L3 A3
  constraint tangent L1 A3
  constraint coincident L5.start L9
  constraint coincident L5.start L1
  constraint tangent L9 A7
  constraint tangent L1 A7
  constraint coincident L4.start L9
  constraint coincident L4.start L7
  constraint tangent L9 A4
  constraint tangent L7 A4
  constraint symmetric L6.start L8 A2.start
  constraint symmetric L0.end L8 A0.end
  constraint symmetric L11.start L16 L17.start
  constraint symmetric L11.end L16 L17.end
  constraint symmetric L12.start L16 L18.start
  constraint symmetric L12.end L16 L18.end
  constraint parallel L4 L19
  constraint midpoint L19.end L20
  constraint vertical L16
  constraint horizontal L8
  constraint midpoint L8 L16.start
  constraint tangent L20 A15
  constraint coincident L12.end L26.start
  constraint coincident L11.end L29.end
  constraint parallel L12 L26
  constraint parallel L11 L29
  constraint horizontal L13
  constraint parallel L0 L15
  constraint parallel L6 L14
  constraint coincident L0 L37.start
  constraint perpendicular L26 L37
  constraint coincident L31 L37.end
  constraint perpendicular L31 L37
  measures "d295" distance of L5.end L4.end
  measures "d296" distance of L4.start L5.end
  measures "d297" radius of A1
  measures "d298" radius of A3
  measures "d299" radius of A7
  measures "d300" radius of A4
  measures "d304" distance of L16.start L13
  measures "d336" vertical distance of L8.end L37.end
extrude "Extrude1''''" add sketch "Sketch1 (4)" along normal mid plane 76 separate body contours A0 L0 L2 A2 L6 L8 L22 L24 A10 L25 A11 | A0 L2 A2 L13 L14 L15 | L0 L8 L12 L15 L26 L31 L37 | L6 L8 L11 L12 L13 L14 L15 L17 L18 L20 L21 L28 L29 L31 L36 L37 makes body 5 in component "Top"
extrude "Extrude10'" cut sketch "Sketch1 (4)" along normal mid plane 74.4 contours A0 L0 L2 A2 L6 L8 L22 L24 A10 L25 A11 bodies 5 in component "Top"
extrude "Extrude3'''" cut sketch "Sketch1 (4)" along normal mid plane 64 contours A0 L2 A2 L13 L14 L15 bodies 5 in component "Top"
sketch "Holes" plane through (0, 0, 0) normal (0, 0, 1) x (1, 0, 0) in component "Top"
  circle A0 centre (-34.5, -6) radius 1
  circle A1 centre (-34.5, -6) radius 2
  circle A2 centre (-34.5, 6) radius 1
  circle A3 centre (-34.5, 6) radius 2
  circle A4 centre (34.5, -6) radius 2
  circle A5 centre (34.5, 6) radius 1
  circle A6 centre (34.5, 6) radius 2
  circle A7 centre (34.5, -6) radius 1
  line L0 (5, -5.5) -> (-19.5, -5.5)
  line L1 (-19.5, -5.5) -> (-19.5, 7.8)
  line L2 (-19.5, 7.8) -> (5, 7.8)
  line L3 (5, 7.8) -> (5, -5.5)
  line L4 (5, -5.5) -> (-19.5, 7.8) construction
  line L5 (-19.5, -5.5) -> (5, 7.8) construction
  circle A8 centre (24, 1.5) radius 6.2
  circle A9 centre (-19.25, -12.75) radius 0.875
  circle A10 centre (-19.25, -12.75) radius 2
  circle A11 centre (-19.25, 11.55) radius 2
  circle A12 centre (-19.25, 11.55) radius 0.875
  circle A13 centre (4.75, -12.75) radius 2
  circle A14 centre (4.75, -12.75) radius 0.875
  circle A15 centre (4.75, 11.55) radius 2
  circle A16 centre (4.75, 11.55) radius 0.875
  point P0 (-34.5, 6)
  point P1 (-34.5, -6)
  point P2 (34.5, 6)
  point P3 (34.5, -6)
  point P4 (-34.5, 6)
  point P5 (34.5, 6)
  point P6 (34.5, -6)
  point P7 (34.5, 6)
  point P8 (-7.25, 1.15)
  point P9 (24, 1.5)
  point P10 (-19.25, -12.75)
  point P11 (4.75, -12.75)
  point P12 (4.75, 11.55)
  point P13 (-19.25, 11.55)
  point P14 (-19.25, 11.55)
  point P15 (4.75, -12.75)
  point P16 (4.75, 11.55)
  dimension "d314" = 2
  dimension "d315" = 4
  dimension "d316" = 2
  dimension "d317" = 4
  dimension "d318" = 2
  dimension "d319" = 4
  dimension "d320" = 2
  dimension "d321" = 4
  dimension "d327" = 24.5
  dimension "d328" = 13.3
  dimension "d329" = 5
  dimension "d330" = 5.5
  dimension "d331" = 12.4
  dimension "d332" = 1.75
  dimension "d333" = 4
  dimension "d343" = 1.75
  dimension "d344" = 4
  dimension "d345" = 1.75
  dimension "d346" = 4
  dimension "d347" = 1.75
  dimension "d348" = 4
  constraint coincident P1 A0.centre
  constraint coincident P4 P0
  constraint coincident P6 P3
  constraint coincident P7 P5
  constraint horizontal L0
  constraint perpendicular L0 L1
  constraint parallel L0 L2
  constraint parallel L1 L3
  constraint coincident L4 P8
  constraint coincident L5 P8
  constraint coincident P9 A8.centre
  constraint coincident P10 A9.centre
  constraint concentric A9 A10
  constraint coincident P14 P13
  constraint concentric A11 A12
  constraint coincident P15 P11
  constraint concentric A13 A14
  constraint coincident P16 P12
  constraint concentric A15 A16
  measures "d314" diameter of A0
  measures "d315" diameter of A1
  measures "d316" diameter of A2
  measures "d317" diameter of A3
  measures "d318" diameter of A7
  measures "d319" diameter of A4
  measures "d320" diameter of A5
  measures "d321" diameter of A6
  measures "d327" distance of L1.end L2.end
  measures "d328" distance of L0.end L1.end
  measures "d329" distance of origin L3
  measures "d330" vertical distance of origin L0.start
  measures "d331" diameter of A8
  measures "d332" diameter of A9
  measures "d333" diameter of A10
  measures "d343" diameter of A12
  measures "d344" diameter of A11
  measures "d345" diameter of A14
  measures "d346" diameter of A13
  measures "d347" diameter of A16
  measures "d348" diameter of A15
extrude "Extrude4''''" cut sketch "Holes" along normal through all contours A0 | A2 | A5 | A7 bodies 5 in component "Top"
extrude "Extrude5''''" cut sketch "Holes" along normal through all from surface at 15.1 contours A1 | A3 | A4 | A6 bodies 5 in component "Top"
chamfer "Chamfer1''" distance 0.5 distance2 1 4 edges at (-35.4323, 5.6384, 15.1) (-35.4323, -6.3616, 15.1) (33.5677, -6.3616, 15.1) (33.5677, 5.6384, 15.1) measured on face at (-33.8018, 6.7159, 14.7667) measured on face at (-33.8018, -5.2841, 14.7667) measured on face at (35.1982, -5.2841, 14.7667) measured on face at (35.1982, 6.7159, 14.7667) on bodies 5 in component "Top"
extrude "Extrude6''" cut sketch "Holes" along normal through all contours L0 L1 L2 L3 | A8 bodies 5 in component "Top"
extrude "Extrude8'" add sketch "Holes" against normal blind 1.5 from surface at 15 contours A10 | A11 | A13 | A15 bodies 5 in component "Top"
extrude "Extrude9'" cut sketch "Holes" against normal blind 4 from surface at 15.6 contours A9 | A12 | A14 | A16 bodies 5 in component "Top"
chamfer "Chamfer2" distance 0.2 distance2 0.2 5 faces at (38, -4, 15.6333) (-38, -4, 15.6333) (1.6667, -11.5536, 16.9) (12.6667, -15.7203, 15.6971) (12.6667, 16.8601, 14.4941) on bodies 5 in component "Top"
sketch "Sketch1 (5)" plane through (0, 0, 0) normal (0, 0, 1) x (1, 0, 0) in component "Knob"
  circle A0 centre (24, 1.5) radius 3
  line L0 (21.3737, 2.95) -> (26.6263, 2.95)
  circle A1 centre (24, 1.5) radius 5
  circle A2 centre (24, 1.5) radius 8.5
  line L1 (24, 1.5) -> (24, 10) construction
  line L2 (24, 1.5) -> (25.1095, 9.9273) construction
  line L3 (24, 1.5) -> (24.5559, 9.9818) construction
  circle A3 centre (24, 10) radius 0.5562
  circle A4 centre (21.8, 9.7104) radius 0.5562
  circle A5 centre (19.75, 8.8612) radius 0.5562
  circle A6 centre (17.9896, 7.5104) radius 0.5562
  circle A7 centre (16.6388, 5.75) radius 0.5562
  circle A8 centre (15.7896, 3.7) radius 0.5562
  circle A9 centre (15.5, 1.5) radius 0.5562
  circle A10 centre (15.7896, -0.7) radius 0.5562
  circle A11 centre (16.6388, -2.75) radius 0.5562
  circle A12 centre (17.9896, -4.5104) radius 0.5562
  circle A13 centre (19.75, -5.8612) radius 0.5562
  circle A14 centre (21.8, -6.7104) radius 0.5562
  circle A15 centre (24, -7) radius 0.5562
  circle A16 centre (26.2, -6.7104) radius 0.5562
  circle A17 centre (28.25, -5.8612) radius 0.5562
  circle A18 centre (30.0104, -4.5104) radius 0.5562
  circle A19 centre (31.3612, -2.75) radius 0.5562
  circle A20 centre (32.2104, -0.7) radius 0.5562
  circle A21 centre (32.5, 1.5) radius 0.5562
  circle A22 centre (32.2104, 3.7) radius 0.5562
  circle A23 centre (31.3612, 5.75) radius 0.5562
  circle A24 centre (30.0104, 7.5104) radius 0.5562
  circle A25 centre (28.25, 8.8612) radius 0.5562
  circle A26 centre (26.2, 9.7104) radius 0.5562
  circle A27 centre (24, 1.5) radius 3.1
  line L4 (21.3153, 3.05) -> (26.6847, 3.05)
  dimension "d356" = 10
  dimension "d357" = 17
  dimension "d358" = 7.5
  dimension "d359" = 3.75
  dimension "d361" = 360
  dimension "d376" = 0.1
  dimension "d377" = 0.1
  constraint concentric A0 A1
  constraint concentric A1 A2
  constraint coincident A0.centre A1.centre
  constraint coincident A2 L1.end
  constraint vertical L1
  constraint coincident A2 L2.end
  constraint coincident A2 L3.end
  constraint coincident L1.end A3.centre
  constraint coincident L3.end A3
  constraint parallel L0 L4
  constraint coincident A27 L4.end
  constraint coincident A27 L4.start
  measures "d356" diameter of A1
  measures "d357" diameter of A2
  measures "d358" angle of L1 L2
  measures "d359" angle of L1 L3
  measures "d377" distance of L0 L4
extrude "Extrude1'''''" add sketch "Sketch1 (5)" along normal blind 7 from surface at 7.9 separate body contours A0 L4 | A0 A27 L4 | A1 picked at (21.5645, 3.2973) makes body 6 in component "Knob"
extrude "Extrude2'''" add sketch "Sketch1 (5)" along normal blind 3 from surface at 14.9 contours A0 L0 | A0 A27 L4 | A0 L0 L4 | A0 L4 | A0 A27 L4 | A1 bodies 6 in component "Knob"
extrude "Extrude3''''" add sketch "Sketch1 (5)" along normal blind 5 from surface at 17.9 contours A0 L0 | A0 A27 L4 | A0 L0 L4 | A0 L4 | A0 A27 L4 | A1 | A2 A3 A4 A5 A6 A7 A8 A9 A10 A11 A12 A13 A14 A15 A16 A17 A18 A19 A20 A21 A22 A23 A24 A25 A26 bodies 6 in component "Knob"
chamfer "Chamfer1'''" distance 0.4 angle 45 1 edges at (19.3384, -0.3081, 17.9) 1 faces at (26.2001, 2.1772, 22.9) on bodies 6 in component "Knob"
chamfer "Chamfer3" distance 0.2 distance2 0.2 3 edges at (19.3384, -0.3081, 7.9) (24, -1.6, 7.9) (24, 3.05, 7.9) measured on face at (28.9752, 1.0022, 11.1) measured on face at (23.6913, -1.5846, 10.2333) measured on face at (23.1051, 3.05, 12.5667) on bodies 6 in component "Knob"
sketch "Sketch1 (6)" plane through (0, 0, 0) normal (1, 0, 0) x (0, 1, 0) in component "Right With Hole (bad)"
  line L0 (12, -13.9) -> (-12, -13.9)
  line L1 (-15, -10.9) -> (-15, 10.9)
  line L2 (-12, 13.9) -> (12, 13.9)
  line L3 (15, 10.9) -> (15, -10.9)
  line L4 (15, -13.9) -> (-15, 13.9) construction
  line L5 (-15, -13.9) -> (15, 13.9) construction
  arc A0 (-12, 13.9) -> (-15, 10.9) centre (-12, 10.9) ccw
  arc A1 (15, 10.9) -> (12, 13.9) centre (12, 10.9) ccw
  arc A2 (12, -13.9) -> (15, -10.9) centre (12, -10.9) ccw
  arc A3 (-15, -10.9) -> (-12, -13.9) centre (-12, -10.9) ccw
  line L6 (-15, -0.9) -> (15, -0.9)
  line L7 (-15, 0.9) -> (15, 0.9)
  arc A4 (13.9, 10.9) -> (12, 12.8) centre (12, 10.9) ccw
  line L8 (-12, 12.8) -> (12, 12.8)
  arc A5 (-12, 12.8) -> (-13.9, 10.9) centre (-12, 10.9) ccw
  line L9 (-13.9, -10.9) -> (-13.9, 10.9)
  arc A6 (-13.9, -10.9) -> (-12, -12.8) centre (-12, -10.9) ccw
  line L10 (12, -12.8) -> (-12, -12.8)
  arc A7 (12, -12.8) -> (13.9, -10.9) centre (12, -10.9) ccw
  line L11 (13.9, 10.9) -> (13.9, -10.9)
  circle A8 centre (-8, -5.65) radius 3.2
  circle A9 centre (-8, -5.65) radius 4.75 construction
  dimension "d192_1" = 30
  dimension "d193_1" = 27.8
  dimension "d194_1" = 3
  dimension "d209_1" = 1.1
  dimension "d393_1" = 1.8
  dimension "d394_1" = 0.9
  dimension "d403" = 6.4
  dimension "d404" = 9.5
  dimension "d405" = 8
  constraint horizontal L0
  constraint perpendicular L0 L1
  constraint parallel L0 L2
  constraint parallel L1 L3
  constraint coincident L4 origin
  constraint coincident L5 origin
  constraint coincident L4.end L1
  constraint coincident L4.end L2
  constraint tangent L1 A0
  constraint tangent L2 A0
  constraint coincident L5.end L3
  constraint coincident L5.end L2
  constraint tangent L3 A1
  constraint tangent L2 A1
  constraint equal A0 A1
  constraint coincident L4.start L0
  constraint coincident L4.start L3
  constraint tangent L0 A2
  constraint tangent L3 A2
  constraint equal A0 A2
  constraint coincident L5.start L0
  constraint coincident L5.start L1
  constraint tangent L0 A3
  constraint tangent L1 A3
  constraint equal A0 A3
  constraint coincident L1 L6.start
  constraint coincident L3 L6.end
  constraint perpendicular L3 L6
  constraint coincident L1 L7.start
  constraint coincident L3 L7.end
  constraint perpendicular L3 L7
  constraint concentric A8 A9
  constraint tangent L6 A9
  measures "d192_1" distance of L4.end L5.end
  measures "d193_1" distance of L5.start L4.end
  measures "d194_1" radius of A0
  measures "d393_1" distance of L6.end L7.end
  measures "d394_1" distance of origin L6
  measures "d403" diameter of A8
  measures "d404" diameter of A9
  measures "d405" horizontal distance of origin A8.centre
extrude "Extrude1''''''" add sketch "Sketch1 (6)" along normal blind 6 from surface at 32 separate body contours L0 L1 L3 A2 A3 L6 L9 A6 L10 A7 L11 | L3 L6 L7 L11 | L1 L6 L7 L9 | L1 L2 L3 A0 A1 L7 A4 L8 A5 L9 L11 | L6 L9 A6 L10 A7 L11 | L6 L7 L9 L11 | L7 A4 L8 A5 L9 L11 | A8 makes body 7 in component "Right With Hole (bad)"
extrude "Extrude2''''" cut sketch "Sketch1 (6)" along normal blind 35 contours L3 L6 L7 L11 | L1 L6 L7 L9 | L6 L7 L9 L11 bodies 7 in component "Right With Hole (bad)"
extrude "Extrude5'''''" cut sketch "Sketch1 (6)" against normal blind 1 from surface at 38 contours L0 L1 L3 A2 A3 L6 L9 A6 L10 A7 L11 | L3 L6 L7 L11 | L1 L6 L7 L9 | L1 L2 L3 A0 A1 L7 A4 L8 A5 L9 L11 bodies 7 in component "Right With Hole (bad)"
extrude "Extrude7'''" cut sketch "Sketch1 (6)" along normal through all contours A8 bodies 7 in component "Right With Hole (bad)"
sketch "Sketch2 (4)" plane through (0, 0, 13.9) normal (0, 0, 1) x (-1, 0, 0) in component "Right With Hole (bad)"
  line L0 (-32, -12) -> (-32, 12)
  line L1 (-32, 12) -> (-37, 12)
  line L2 (-37, -12) -> (-32, -12)
  line L3 (0, 0) -> (-32, 0) construction
  line L4 (-32, 0) -> (-37, 0) construction
  line L5 (-34.5, 0) -> (-34.5, -6) construction
  circle A0 centre (-34.5, -6) radius 0.875
  circle A1 centre (-34.5, 6) radius 0.875
  line L6 (-37, 12) -> (-37, -12)
  dimension "d202_1" = 6
  dimension "d203_1" = 1.75
  constraint coincident L3.start origin
  constraint midpoint L0 L3.end
  constraint midpoint L4 L5.start
  constraint perpendicular L4 L5
  constraint coincident L5.end A0.centre
  constraint symmetric L4 A0 A1
  constraint midpoint L4.end L6
  measures "d202_1" distance of L5.start L5.end
  measures "d203_1" diameter of A0
extrude "Extrude3'''''" cut sketch "Sketch2 (4)" against normal blind 4 contours A0 | A1 bodies 7 in component "Right With Hole (bad)"
extrude "Extrude4'''''" cut sketch "Sketch2 (4)" along normal blind 4 from surface at -27.8 contours A0 | A1 bodies 7 in component "Right With Hole (bad)"
chamfer "Chamfer1''''" distance 0.2 angle 45 10 edges at (37, 0, 13.9) (37, 14.1213, 13.0213) (37, 15, 0) (37, 14.1213, -13.0213) (37, 0, -13.9) (37, -14.1213, -13.0213) (37, -15, 0) (37, -14.1213, 13.0213) (38, -10.9834, -4.4928) (32, -10.9834, -6.8072) 2 faces at (32, -4, 5.2333) (32, 7.4, -6.8167) on bodies 7 in component "Right With Hole (bad)"
component "Board" placed x (1, 0, 0) y (0, 1, 0) z (0, 0, 1) at (0, 0, 0)
component "Right" placed x (1, 0, 0) y (0, 1, 0) z (0, 0, 1) at (0, 0, 0)
component "Left" placed x (1, 0, 0) y (0, 1, 0) z (0, 0, 1) at (0, 0, 0)
component "Bottom" placed x (1, 0, 0) y (0, 1, 0) z (0, 0, 1) at (0, 0, 0)
component "Top" placed x (1, 0, 0) y (0, 1, 0) z (0, 0, 1) at (0, 0, 0)
component "Knob" placed x (1, 0, 0) y (0, 1, 0) z (0, 0, 1) at (0, 0, 0)
component "Right With Hole (bad)" placed x (1, 0, 0) y (0, 1, 0) z (0, 0, 1) at (0, 0, 0)
hidden bodies 1
equation "d8 = 70 mm - 2 mm - 2 mm"
equation "d9 = 30 mm - 2 mm - 2 mm"
equation "d55 = ( 7 * 2.54 ) * 1 mm"
equation "d193 = 13 mm * 2 + d393"
equation "d197 = ( ( 70 / 2 ) * 1 mm ) - 3 mm"
equation "d200 = ( 70 / 2 ) * 1 mm"
equation "d215 = ( 13 * 2 ) * 1 mm + d395"
equation "d218 = d395 / 2"
equation "d223 = -( ( 70 / 2 ) * 1 mm - 3 mm )"
equation "d226 = -( ( 70 / 2 ) * 1 mm )"
equation "d245 = ( 13 * 2 ) * 1 mm + 1.8 mm"
equation "d253 = ( 70 / 2 ) * 1 mm - 3 mm + 6 mm"
equation "d261 = ( 70 / 2 ) * 1 mm - 3 mm + 6 mm - 1 mm + 0.2 mm"
equation "d285 = ( 70 / 2 ) * 1 mm - 3 mm"
equation "d296 = ( 13 * 2 ) * 1 mm + 1.8 mm"
equation "d308 = ( 70 / 2 ) * 1 mm - 3 mm + 6 mm"
equation "d312 = ( 70 / 2 ) * 1 mm - 3 mm"
equation "d358 = ( 360 / 24 / 2 ) * 1 deg"
equation "d359 = d358 / 2"
equation "d393 = 1.6 mm + 0.2 mm"
equation "d394 = d393 / 2"
equation "d398 = ( 70 / 2 ) * 1 mm - 3 mm + 6 mm - 1 mm + 0.2 mm"
equation "d400 = ( ( 30 - 10 * 2.54 ) / 2 ) * 1 mm"
equation "d402 = d400"
equation "d193_1 = 13 mm * 2 + d393_1"
equation "d197_1 = ( ( 70 / 2 ) * 1 mm ) - 3 mm"
equation "d200_1 = ( 70 / 2 ) * 1 mm"